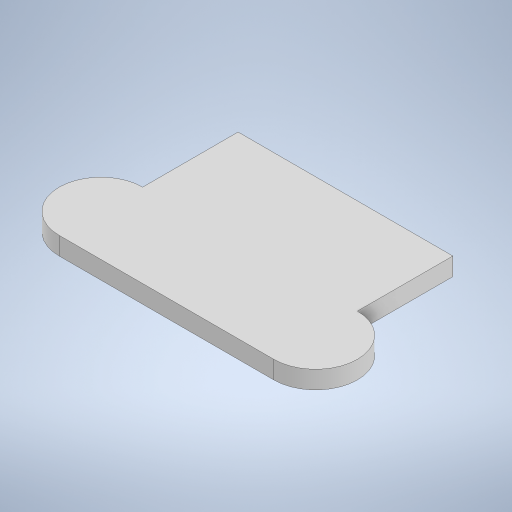
# Autodesk Inventor part: reset
Saved by Autodesk Inventor 2024.1 (Build 281209000, 209)
## iProperties
Created: 2025-04-13
Part Number: reset
Material: 一般
Document SubType Name: Modeling
Designer: hibik
Density: 1 g/cm^3
Appearance: 既定
Author: hibik
Autodesk Inventor part; units mm, degrees
ref_plane "YZ Plane" through (0, 0, 0) normal (1, 0, 0) x (0, 1, 0)
ref_plane "XZ Plane" through (0, 0, 0) normal (0, 1, 0) x (-1, 0, 0)
ref_plane "XY Plane" through (0, 0, 0) normal (0, 0, 1) x (1, 0, 0)
sketch "スケッチ1" plane through (0, 0, 0) normal (0, 1, 0) x (-1, 0, 0)
  line L0 (0, 0) -> (25, 0)
  line L1 (25, 0) -> (25, -15)
  line L2 (25, -15) -> (0, -15)
  line L3 (0, -15) -> (0, 0)
  circle A0 centre (21.5, -3.5) radius 3.5
  circle A1 centre (3.5, -3.5) radius 3.5
  line L4 (21.5, -3.5) -> (21.5, -15)
  line L5 (3.5, -3.5) -> (3.5, -15)
  point P0 (21.5, 0)
  point P1 (3.5, 0)
  point P2 (3.5, -7)
  point P3 (21.5, -7)
  dimension "d0" = 25
  dimension "d1" = 15
  dimension "d2" = 7
  dimension "d3" = 7
  constraints: 12 end point, 4 tangent, 3 perpendicular, 2 centre point, 2 parallel, 2 point on line, 1 horizontal
  measures "d0" distance of L1.end L2.end
  measures "d1" distance of L0.end L1.end
  measures "d2" diameter of A0
  measures "d3" diameter of A1
extrude "押し出し1" add sketch "スケッチ1" along normal blind 1.5 contours L0 A0 L4 L2 L5 A1 | A1 | A0
